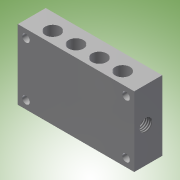
# Autodesk Inventor part: Manifold_v5
Saved by Autodesk Inventor 2016 (Build 200138000, 138)
## iProperties
Created: 2015-03-09
Part Number: Manifold_v5
Material: Generic
Document SubType Name: Modeling
Designer: User
Density: 1 g/cm^3
Appearance: Steel
Author: User
Autodesk Inventor part; units mm, degrees
sketch "Sketch1" plane through (0, 0, 0) normal (1, 0, 0) x (0, 1, 0)
  line L0 (0, 0) -> (12, 0)
  line L1 (12, 0) -> (12, -30)
  line L2 (12, -30) -> (0, -30)
  line L3 (0, -30) -> (0, 0)
  circle A0 centre (5, -15) radius 0.4
  dimension "d0" = 30
  dimension "d1" = 12
  dimension "d2" = 5
  dimension "d3" = 15
  dimension "d4" = 0.8
  constraints: 8 end point, 2 parallel, 1 centre point, 1 horizontal, 1 perpendicular
  measures "d0" distance of L0.end L1.end
  measures "d1" distance of L1.end L2.end
  measures "d2" distance from line of L3 A0.centre
  measures "d3" distance from line of L0 A0.centre
  measures "d4" diameter of A0
extrude "Extrusion1" add sketch "Sketch1" against normal blind 50
ref_plane "Work Plane1" through (0, 0, -15) normal (0, 0, 1) x (1, 0, 0)
sketch "Sketch2" plane through (0, 0, 0) normal (0, 0, 1) x (1, 0, 0)
  line L0 (0, 0) -> (-50, 0) projected
  line L1 (0, 0) -> (0, 12) projected
  circle A0 centre (-10, 5) radius 3.2
  dimension "d7" = 6.4
  dimension "d8" = 5
  dimension "d9" = 10
  constraints: 1 centre point
  measures "d7" diameter of A0
  measures "d8" distance from line of L0 A0.centre
  measures "d9" distance from line of L1 A0.centre
extrude "Extrusion4" cut sketch "Sketch2" against normal blind 10.8
pattern_linear "Rectangular Pattern1" count 4 spacing 10 along (-1, 0, 0) of "Extrusion4"
ref_plane "Work Plane2" through (0, 5, -14.6) normal (0, 0, 1) x (1, 0, 0)
sketch "Sketch3" plane through (-10, 5, -10.8) normal (0, 0, 1) x (1, 0, 0)
  circle A0 centre (0, 0) radius 0.4
  circle A1 centre (0, 0) radius 3.2 projected
  point P0 (10, -5)
  dimension "d20" = 0.8
  constraints: 1 centre point, 1 concentric
  measures "d20" diameter of A0
extrude "Extrusion5" cut sketch "Sketch3" against normal blind 10 contours A0
pattern_linear "Rectangular Pattern2" count 4 spacing 10 along (-1, 0, 0) of "Extrusion5"
ref_plane "Work Plane3" through (0, 6, -30) normal (0, -1, 0) x (1, 0, 0)
sketch "Sketch4" plane through (0, 12, 0) normal (0, 1, 0) x (1, 0, 0)
  line L0 (0, 0) -> (0, 30) projected
  line L1 (0, 0) -> (-50, 0) projected
  circle A0 centre (-10, 7.25) radius 0.4
  circle A1 centre (-3.5, 3.5) radius 1.6
  dimension "d26" = 0.8
  dimension "d27" = 7.25
  dimension "d28" = 10
  dimension "d93" = 3.2
  dimension "d94" = 3.5
  dimension "d95" = 3.5
  constraints: 2 centre point
  measures "d26" diameter of A0
  measures "d27" distance from line of L1 A0.centre
  measures "d28" distance from line of L0 A0.centre
  measures "d93" diameter of A1
  measures "d94" distance from line of L1 A1.centre
  measures "d95" distance from line of L0 A1.centre
hole "Hole1" at (-10, 12, -7.25) direction (0, -1, 0) diameter 2.46 depth 7 thread size "M3x0.5" class "6H" standard "ANSI Metric M Profile"
pattern_linear "Rectangular Pattern4" count 4 spacing 10 along (-1, 0, 0) count 2 spacing 15.2 along (0, 0, -1) of "Hole1"
sketch "Sketch5" plane through (0, 0, -30) normal (0, 0, -1) x (-1, 0, 0)
  circle A0 centre (10, 5) radius 3.2
  line L0 (0, 12) -> (50, 12) projected
  line L1 (0, 12) -> (0, 0) projected
  line L2 (0, 0) -> (50, 0) projected
  dimension "d47" = 6.4
  dimension "d49" = 10
  dimension "d109" = 5
  constraints: 1 centre point
  measures "d47" diameter of A0
  measures "d49" distance from line of L1 A0.centre
  measures "d109" distance from line of L2 A0.centre
hole "Hole2" at (-10, 5, -30) direction (0, 0, 1) diameter 6.3 depth 10.8
pattern_linear "Rectangular Pattern5" count 4 spacing 10 along (-1, 0, 0) of "Hole2", "Extrusion4"
hole "Hole3" at (0, 5, -15) direction (-1, 0, 0) diameter 5.36 depth 7 thread size "1/4-28 UNF" class "2B" standard "ANSI Unified Screw Threads"
sketch "Sketch6" plane through (-50, 0, 0) normal (-1, 0, 0) x (0, 0, 1)
  circle A0 centre (-15, 5) radius 2.15
  line L0 (-30, 0) -> (0, 0) projected
  dimension "d67" = 15
  dimension "d68" = 5
  dimension "d69" = 4.3
  constraints: 1 centre point
  measures "d67" horizontal distance of L0.end A0.centre
  measures "d68" distance from line of L0 A0.centre
  measures "d69" diameter of A0
hole "Hole4" at (-50, 5, -15) direction (1, 0, 0) diameter 5.36 depth 7 thread size "1/4-28 UNF" class "2B" standard "ANSI Unified Screw Threads"
hole "Hole5" at (-3.5, 12, -3.5) direction (0, -1, 0) diameter 3.2 end through all
pattern_linear "Rectangular Pattern6" count 2 spacing 43 along (-1, 0, 0) count 2 spacing 23 along (0, 0, -1) of "Hole5"
equation "\"d3\" = 0.5 * d0"
body "Solid1"
